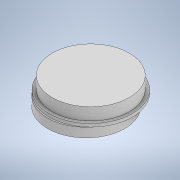
# Autodesk Inventor part: Motor_to_gearbox
Saved by Autodesk Inventor 2021 (Build 250183000, 183)
## iProperties
Created: 2022-08-30
Part Number: Motor_to_gearbox
Material: Ogólny
Document SubType Name: Modeling
Designer: MicnedSQ
Density: 1 g/cm^3
Appearance: Domyślna
Author: MicnedSQ
Autodesk Inventor part; units mm, degrees
ref_plane "YZ Plane" through (0, 0, 0) normal (1, 0, 0) x (0, 1, 0)
ref_plane "XZ Plane" through (0, 0, 0) normal (0, 1, 0) x (-1, 0, 0)
ref_plane "XY Plane" through (0, 0, 0) normal (0, 0, 1) x (1, 0, 0)
sketch "Szkic1" plane through (0, 0, 0) normal (0, 1, 0) x (-1, 0, 0)
  circle A0 centre (0, 0) radius 12.5
  dimension "d0" = 25
  constraints: 1 centre point, 1 coincident
  measures "d0" diameter of A0
extrude "Wyciągnięcie proste1" add sketch "Szkic1" along normal blind 3
sketch "Szkic4" plane through (0, 3, 0) normal (0, 1, 0) x (1, 0, 0)
  circle A0 centre (0, 1.5) radius 13.5
  point P0 (0, 0)
  dimension "d7" = 27
  constraints: 1 centre point
  measures "d7" diameter of A0
extrude "Wyciągnięcie proste3" add sketch "Szkic4" along normal blind 1
sketch "Szkic5" plane through (0, 4, -1.5) normal (0, 1, 0) x (1, 0, 0)
  circle A0 centre (0, 0) radius 12.5
  point P0 (0, -1.5)
  dimension "d10" = 25
  constraints: 1 centre point
  measures "d10" diameter of A0
extrude "Wyciągnięcie proste4" add sketch "Szkic5" along normal blind 4
